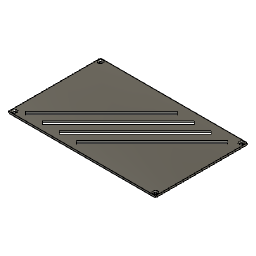
module_lid v3 (Autodesk Fusion 360 design; units mm, degrees)
Autodesk Fusion 360 part; units mm, degrees
sketch "Sketch1" plane through (0, 0, 0) normal (0, 0, 1) x (1, 0, 0)
  line L0 (0, 0) -> (174, 0)
  line L1 (174, 0) -> (174, 109)
  line L2 (174, 109) -> (0, 109)
  line L3 (0, 109) -> (0, 0)
  dimension "d1" = 174
  dimension "d2" = 109
  constraint horizontal L0
  constraint vertical L1
  constraint horizontal L2
  constraint vertical L3
  constraint coincident L0.start L3.end
  measures "d1" distance of L0.start L0.end
  measures "d2" distance of L0.start L2.end
extrude "Extrude1" add sketch "Sketch1" along normal blind 2
sketch "Sketch2" plane through (0, 0, 2) normal (0, 0, 1) x (-1, 0, 0)
  line L0 (0, -109) -> (0, 0)
  line L1 (0, 0) -> (-174, 0)
  line L2 (-174, 0) -> (-174, -109)
  line L3 (-174, -109) -> (0, -109)
  point P0 (-3.5, -3.5)
  point P1 (-3.5, -105.5)
  point P2 (-170.5, -105.5)
  point P3 (-170.5, -3.5)
hole "Hole1" at (170.5, 3.5, 2) at (3.5, 105.5, 2) at (3.5, 3.5, 2) at (170.5, 105.5, 2) direction (0, 0, -1) diameter 3.4 depth 6 tip angle 180 countersink diameter 5.75 countersink angle 90
sketch "Sketch5" plane through (0, 0, 2) normal (0, 0, 1) x (-1, 0, 0)
  circle A0 centre (-3.5, -3.5) radius 2.875
  circle A1 centre (-170.5, -3.5) radius 2.875
  circle A2 centre (-3.5, -105.5) radius 2.875
  circle A3 centre (-170.5, -105.5) radius 2.875
  line L0 (0, -109) -> (0, 0)
  line L1 (0, 0) -> (-174, 0)
  line L2 (-174, 0) -> (-174, -109)
  line L3 (-174, -109) -> (0, -109)
  line L4 (-10, -10) -> (-100, -100)
  line L5 (-100, -100) -> (-103.5355, -96.4645)
  line L6 (-103.5355, -96.4645) -> (-13.5355, -6.4645)
  line L7 (-13.5355, -6.4645) -> (-10, -10)
  line L8 (-30, -10) -> (-120, -100)
  line L9 (-123.5355, -96.4645) -> (-33.5355, -6.4645)
  line L10 (-33.5355, -6.4645) -> (-30, -10)
  line L11 (-120, -100) -> (-123.5355, -96.4645)
  line L12 (-50, -10) -> (-140, -100)
  line L13 (-143.5355, -96.4645) -> (-53.5355, -6.4645)
  line L14 (-53.5355, -6.4645) -> (-50, -10)
  line L15 (-140, -100) -> (-143.5355, -96.4645)
  line L16 (-70, -10) -> (-160, -100)
  line L17 (-163.5355, -96.4645) -> (-73.5355, -6.4645)
  line L18 (-73.5355, -6.4645) -> (-70, -10)
  line L19 (-160, -100) -> (-163.5355, -96.4645)
  dimension "d17" = 5
  dimension "d20" = -60
  dimension "d21" = 0
  constraint perpendicular L4 L5
  constraint parallel L4 L6
  constraint parallel L5 L7
  measures "d17" distance of L4.start L6.end
extrude "Extrude2" cut sketch "Sketch5" against normal blind 40 contours L4 L5 L6 L7 | L8 L9 L10 L11 | L12 L13 L14 L15 | L16 L17 L18 L19
